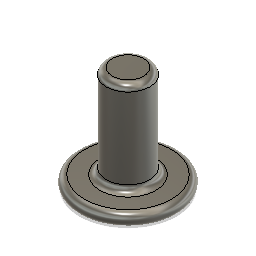
ball-ejector (Autodesk Fusion 360 design; units mm, degrees)
Autodesk Fusion 360 part; units mm, degrees
sketch "スケッチ1" plane through (0, 0, 0) normal (0, 1, 0) x (1, 0, 0)
  circle A0 centre (0, 0) radius 3.5
  circle A1 centre (0, 0) radius 8
  dimension "d1" = 7
  dimension "d14" = 16
  constraint coincident A0.centre A1.centre
  measures "d1" diameter of A0
  measures "d14" diameter of A1
extrude "押し出し1" add sketch "スケッチ1" along normal blind 15 contours A0 makes body 1
extrude "押し出し2" add sketch "スケッチ1" against normal blind 2 contours A0 | A1 bodies 1
sphere "球プリミティブ1" add diameter 34 placed x (1, 0, 0) y (0, 0, -1) z (0, 1, 0) at (0, 0, 0) separate body makes body 2
move_body "移動1" bodies 2 to x (1, 0, 0) y (0, 1, 0) z (0, 0, 1) at (0, 38.5, 0)
fillet "フィレット4" radius 1 1 edges at (-3.2631, 0, 1.2657) on bodies 1
fillet "フィレット5" radius 1 1 edges at (-3.2631, 15, 1.2657) on bodies 1
fillet "フィレット6" radius 1 2 edges at (-7.4586, 0, 2.8929) (-7.4586, -2, -2.8929) on bodies 1
delete_body "RemoveBody1" bodies 2
